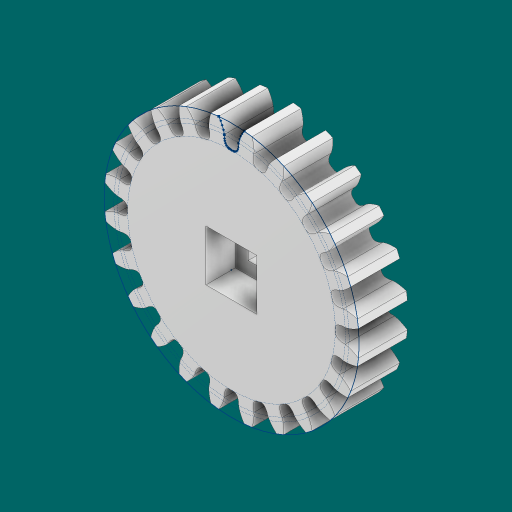
# Autodesk Inventor part: motor_pinion
Saved by Autodesk Inventor 2023.1 (Build 271208000, 208)
## iProperties
Created: 2022-11-06
Part Number: motor_pinion
Material: ABS Plastic
Document SubType Name: Modeling
Designer: zac-h
Density: 1.06 g/cm^3
Appearance: Smooth - White
Author: zac-h
## iProperties of the stored document motor_pinion_3DPrint.ipt
Created: 2022-11-06
Part Number: motor_pinion_3DPrint
Material: Generic
Document SubType Name: Modeling
Designer: zac-h
Density: 1 g/cm^3
Appearance: Default
Author: zac-h
Autodesk Inventor part; units mm, degrees
ref_plane "YZ Plane" through (0, 0, 0) normal (1, 0, 0) x (0, 1, 0)
ref_plane "XZ Plane" through (0, 0, 0) normal (0, 1, 0) x (-1, 0, 0)
ref_plane "XY Plane" through (0, 0, 0) normal (0, 0, 1) x (1, 0, 0)
sketch "Sketch1" plane through (0, 0, 0) normal (0, 0, 1) x (1, 0, 0)
  spline S0 degree 3 poles (-1.6482, 16.4275) (-1.5683, 16.2966) (-1.4084, 16.0347) (-1.2058, 15.6216) (-1.0298, 15.1951) (-0.9667, 14.8946) (-0.9351, 14.7444) knots 0 0 0 0 0.045995 0.091986 0.13797 0.183904 0.183904 0.183904 0.183904
  spline S1 degree 3 poles (-0.9351, 14.7444) (-0.9349, 14.588) (-0.9345, 14.3532) (-0.8763, 14.0449) (-0.7935, 13.8247) (-0.6625, 13.6266) (-0.4997, 13.512) (-0.3522, 13.4571) (-0.1949, 13.4489) (0, 13.4554) (0.1949, 13.4489) (0.3522, 13.4571) (0.4997, 13.512) (0.6625, 13.6266) (0.7935, 13.8247) (0.8763, 14.0449) (0.9345, 14.3532) (0.9349, 14.588) (0.9351, 14.7444) knots 0 0 0 0 0.046825 0.07026 0.093695 0.117049 0.140365 0.152081 0.163794 0.187233 0.210673 0.222386 0.234102 0.257418 0.280772 0.304206 0.327642 0.374466 0.374466 0.374466 0.374466
  spline S2 degree 3 poles (0.9351, 14.7444) (0.9667, 14.8946) (1.0298, 15.1951) (1.2058, 15.6216) (1.4084, 16.0347) (1.5683, 16.2966) (1.6482, 16.4275) knots 0 0 0 0 0.045934 0.091918 0.137909 0.183904 0.183904 0.183904 0.183904
  circle A0 centre (0, 0) radius 13.4528 construction
  circle A1 centre (0, 0) radius 14.7546 construction
  circle A2 centre (0, 0) radius 15.24 construction
  circle A3 centre (0, 0) radius 16.51
  point P0 (-1.4146, 16.0313)
  point P1 (-1.2102, 15.6193)
  point P2 (-1.0433, 15.1909)
  point P3 (-0.9151, 14.2766)
  point P4 (-0.8698, 14.0467)
  point P5 (-0.7853, 13.8281)
  point P6 (-0.6517, 13.6366)
  point P7 (-0.4617, 13.5014)
  point P8 (-0.351, 13.4629)
  point P9 (-0.2344, 13.452)
  point P10 (0, 13.4528)
  point P11 (0.2344, 13.452)
  point P12 (0.351, 13.4629)
  point P13 (0.4617, 13.5014)
  point P14 (0.6517, 13.6366)
  point P15 (0.7853, 13.8281)
  point P16 (0.8698, 14.0467)
  point P17 (0.9151, 14.2766)
  point P18 (1.0433, 15.1909)
  point P19 (1.2102, 15.6193)
  point P20 (1.4146, 16.0313)
  constraints: 4 centre point, 2 point on circle, 57 other
extrude "Extrusion1" add sketch "Sketch1" against normal blind 6.35
extrude "Extrusion2" cut sketch "Sketch1" against normal through all contours A3 S2 S1 S0 picked at (0.1985, 15.6803)
pattern_circular "Circular Pattern1" count 24 over 360 about axis through (0, 0, 0) along (0, 0, -1) of "Extrusion2"
sketch "Sketch2" plane through (0, 0, 0) normal (0, 0, 1) x (1, 0, 0)
  line L0 (-3.302, -3.302) -> (3.302, -3.302)
  line L1 (3.302, -3.302) -> (3.302, 3.302)
  line L2 (3.302, 3.302) -> (-3.302, 3.302)
  line L3 (-3.302, 3.302) -> (-3.302, -3.302)
  line L4 (-3.302, -3.302) -> (3.302, 3.302) construction
  line L5 (3.302, -3.302) -> (-3.302, 3.302) construction
  point P0 (0, 0)
  dimension "d7" = 6.604
  dimension "d8" = 6.604
  constraints: 12 end point, 2 midpoint, 2 parallel, 1 horizontal, 1 perpendicular
  measures "d7" distance of L2.end L1.end
  measures "d8" distance of L1.end L0.end
extrude "Extrusion3" cut sketch "Sketch2" against normal blind 3.81
sketch "Sketch3" plane through (0, 0, -3.81) normal (0, 0, 1) x (1, 0, 0)
  line L0 (-1.651, -1.651) -> (1.651, -1.651)
  line L1 (1.651, -1.651) -> (1.651, 1.651)
  line L2 (1.651, 1.651) -> (-1.651, 1.651)
  line L3 (-1.651, 1.651) -> (-1.651, -1.651)
  line L4 (-1.651, -1.651) -> (1.651, 1.651) construction
  line L5 (1.651, -1.651) -> (-1.651, 1.651) construction
  point P0 (0, 0)
  dimension "d11" = 3.302
  dimension "d12" = 3.302
  constraints: 12 end point, 2 midpoint, 2 parallel, 1 horizontal, 1 perpendicular
  measures "d11" distance of L2.end L1.end
  measures "d12" distance of L1.end L0.end
extrude "Extrusion4" cut sketch "Sketch3" against normal through all
equation "\"d0\" = FaceWidth"
equation "\"Module\" = 1.27"
equation "\"PressureAngle\" = 14.5deg"
equation "\"UnitProfileClearance\" = 0.25"
equation "\"UnitRoundRadius\" = 0.3335"
equation "\"HeadDiameter\" = 33.02"
equation "\"RootDiameter\" = 26.90561"
equation "\"BaseDiameter\" = 29.50914"
equation "\"PitchDiameter\" = 30.48"
equation "\"FaceWidth\" = 6.35"
equation "\"HelixAngle\" = 0"
equation "\"UnitCorrection\" = 0"
equation "\"UnitAddendumModification\" = 0"
equation "\"CircularPitch\" = 3.98982"
equation "\"UnitBacklashShift\" = -0.157241"
equation "\"TotalToolShift\" = -0.1997"
equation "\"IsInternal\" = 0"
body "Solid1"
